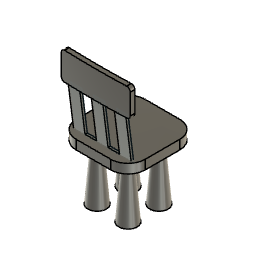
Chair (Autodesk Fusion 360 design; units mm, degrees)
Autodesk Fusion 360 part; units mm, degrees
note: some values were not read from the file. Chosen so that the rebuilt part matches the saved one: which face or edge a step refers to. Set by a fixed rule: which sketch regions a step uses.
sketch "Sketch1" plane through (0, 0, 0) normal (0, 0, 1) x (1, 0, 0)
  line L0 (0, 0) -> (20, 0)
  line L1 (0, 0) -> (0, 250)
  spline S0 degree 5 poles (0, 250) (1.763, 249.8564) (5.2208, 249.5461) (10.2027, 249.0117) (16.4289, 248.1586) (23.4627, 246.8396) (29.6575, 245.2376) (34.2312, 243.5585) (37.1499, 242.0595) (38.8803, 240.8979) (39.7703, 240.1911) (40, 240) knots 0 0 0 0 0 0 0.1 0.2 0.3 0.4 0.5 0.6 0.63638 0.63638 0.63638 0.63638 0.63638 0.63638
  line L2 (20, 0) -> (40, 240)
  dimension "d4" = 250
  dimension "d6" = 20
  constraint coincident L0.start L1.start
  constraint perpendicular L0 L1
  measures "d4" distance of L0.start L1.end
  measures "d6" distance of L0.start L0.end
revolve "Revolve1" add sketch "Sketch1" angle 360 about axis through (0, 0, 0) along (0, 1, 0) makes body 1
move_body "Move1" bodies 1 to x (1, 0, 0) y (0, 0, -1) z (0, 1, 0) at (0, 25, 250)
ref_plane "WorkPlane1" through (0, 120, 0) normal (0, 1, 0) x (0, 0, 1)
sketch "Sketch2" plane through (0, 120, 0) normal (0, 1, 0) x (1, 0, 0)
pattern_circular "C-Pattern1" count 4 over 360 about axis through (0, 120, 0) along (0, 0, 1) of bodies 1 makes body 2 at (78.3678, 154.5371, 30) makes body 3 at (-34.5371, 198.3678, 30) makes body 4 at (-68.9267, 91.8997, 30)
sketch "Sketch3" plane through (0, 0, 250) normal (0, 0, 1) x (-1, 0, 0)
  circle A0 centre (0, -215) radius 20
  line L0 (106.1582, -225.9737) -> (0.1845, -332.132)
  line L1 (106.1582, -225.9737) -> (212.132, -119.8155)
  line L2 (212.132, -119.8155) -> (-0.1845, 92.132)
  line L3 (-0.1845, 92.132) -> (-212.132, -120.1845)
  line L4 (-212.132, -120.1845) -> (0.1845, -332.132)
  constraint perpendicular L1 L2
  constraint perpendicular L2 L3
  constraint perpendicular L0 L4
extrude "Extrude1" add sketch "Sketch3" along normal blind 40 contours A0 | L0 L1 L2 L3 L4 bodies 1 2 3 4
fillet "Fillet1" radius 75 1 edges at (0.1845, -92.132, 270) on bodies 1
fillet "Fillet2" radius 75 1 edges at (212.132, 120.1845, 270) on bodies 1
fillet "Fillet3" radius 75 1 edges at (-0.1845, 332.132, 270) on bodies 1
fillet "Fillet4" radius 75 1 edges at (-212.132, 119.8155, 270) on bodies 1
ref_plane "WorkPlane2" through (88.4652, 31.6886, 270) normal (0.707722, -0.706491, 0) x (0.706491, 0.707722, 0)
sketch "Sketch4" plane through (28.4653, -28.4158, 0) normal (0.707722, -0.706491, 0) x (0.706491, 0.707722, 0)
  line L0 (-65, 275) -> (-25, 275)
  line L1 (-25, 275) -> (-15, 275)
  line L2 (-15, 275) -> (-25, 275)
  line L3 (-25, 275) -> (-50, 470)
  line L4 (-50, 470) -> (-40, 470)
  line L5 (-40, 470) -> (-15, 275)
  dimension "d25" = 40
  dimension "d26" = 10
  dimension "d27" = 10
  constraint horizontal L0
  constraint parallel L0 L1
  constraint horizontal L2
  constraint horizontal L4
  measures "d25" distance of L0.start L0.end
  measures "d26" distance of L0.end L1.end
  measures "d27" distance of L1.end L0.end
extrude "Extrude2" add sketch "Sketch4" against normal blind 250 separate body makes body 5
ref_plane "WorkPlane3" through (-79.4284, 40.4333, 372.5) normal (0.700756, 0.701976, 0.127164) x (0.08984, 0.089997, -0.991882)
sketch "Sketch5" plane through (14.0796, 14.1041, 2.555) normal (0.700756, 0.701976, 0.127164) x (0.08984, 0.089997, -0.991882)
ref_plane "WorkPlane4" through (0, 120, 290) normal (0, 0, 1) x (1, 0, 0)
sketch "Sketch6" plane through (0, 0, 290) normal (0, 0, 1) x (1, 0, 0)
move_body "Move2" bodies 5 1 to x (0.707107, 0.707107, 0) y (-0.707107, 0.707107, 0) z (0, 0, 1) at (84.8528, 35.1472, 0)
sketch "Sketch7" plane through (0, 0, 290) normal (0, 0, 1) x (-1, 0, 0)
  arc A0 (149.9347, -44.8695) -> (74.8695, 30.0652) centre (74.9347, -44.9348) ccw
  line L0 (74.8695, 30.0652) -> (-75.1305, 29.9347)
  arc A1 (-75.1305, 29.9347) -> (-150.0652, -45.1305) centre (-75.0652, -45.0653) ccw
  line L1 (-150.0652, -45.1305) -> (-149.9347, -195.1305)
  arc A2 (-149.9347, -195.1305) -> (-74.8695, -270.0652) centre (-74.9347, -195.0652) ccw
  line L2 (-74.8695, -270.0652) -> (75.1305, -269.9347)
  arc A3 (75.1305, -269.9347) -> (150.0652, -194.8695) centre (75.0652, -194.9347) ccw
  line L3 (150.0652, -194.8695) -> (149.9347, -44.8695)
  line L4 (-125, -50) -> (-75, -49.9565)
  line L5 (-75, -49.9565) -> (-25, -49.913)
  line L6 (-25, -49.913) -> (24.9999, -49.8695)
  line L7 (24.9999, -49.8695) -> (74.9999, -49.826)
  line L8 (74.9999, -49.826) -> (124.9999, -49.7825)
  line L9 (-75, -49.9565) -> (-25, -49.9565)
  line L10 (-25, -49.9565) -> (-25, 21.5768)
  line L11 (-25, 21.5768) -> (-75, 21.5768)
  line L12 (-75, 21.5768) -> (-75, -49.9565)
  line L13 (24.9999, -49.8695) -> (74.9999, -49.8695)
  line L14 (74.9999, -49.8695) -> (74.9999, 17.9113)
  line L15 (74.9999, 17.9113) -> (24.9999, 17.9113)
  line L16 (24.9999, 17.9113) -> (24.9999, -49.8695)
  dimension "d44" = 50
  dimension "d45" = 50
  dimension "d46" = 50
  dimension "d47" = 50
  dimension "d48" = 50
  dimension "d49" = 50
  dimension "d50" = 50
  constraint perpendicular L1 L4
  constraint parallel L4 L5
  constraint parallel L5 L6
  constraint parallel L5 L7
  constraint parallel L7 L8
  constraint horizontal L9
  constraint vertical L10
  constraint horizontal L11
  constraint vertical L12
  constraint horizontal L13
  constraint vertical L14
  constraint horizontal L15
  constraint vertical L16
  measures "d44" distance of L4.start L4.end
  measures "d45" distance of L4.end L5.end
  measures "d46" distance of L5.end L6.end
  measures "d47" distance of L6.end L7.end
  measures "d48" distance of L7.end L8.end
  measures "d49" distance of L4.end L9.end
  measures "d50" distance of L6.end L13.end
extrude "Extrude3" cut sketch "Sketch7" along normal blind 195 contours L5 L10 L11 L12 | L7 L14 L15 L16 bodies 5
sketch "Sketch8" plane through (-0.0474, 54.435, 6.9789) normal (-0.000863, 0.991881, 0.127164) x (-1, -0.00087, 0)
  line L0 (-24.9957, 466.8109) -> (-25.0158, 285.3376)
  line L1 (-25.0158, 285.3376) -> (-75.0158, 285.3376)
  line L2 (-75.0158, 285.3376) -> (-74.9958, 466.8109)
  line L3 (-74.9958, 466.8109) -> (-125.1044, 466.8109)
  line L4 (-125.1044, 466.8109) -> (-125.1044, 270.2148)
  line L5 (-125.1044, 270.2148) -> (124.8956, 270.2148)
  line L6 (124.8956, 270.2148) -> (124.8956, 466.8109)
  line L7 (124.8956, 466.8109) -> (75.0043, 466.8109)
  line L8 (75.0043, 466.8109) -> (74.9842, 285.3376)
  line L9 (74.9842, 285.3376) -> (24.9842, 285.3376)
  line L10 (24.9842, 285.3376) -> (25.0042, 466.8109)
  line L11 (25.0042, 466.8109) -> (-24.9957, 466.8109)
sketch "Sketch9" plane through (0, 0, 470) normal (0, 0, 1) x (-1, 0, 0)
  line L0 (-25, 14.9049) -> (-25, 4.9049)
  line L1 (-25, 4.9049) -> (24.9999, 4.9484)
  line L2 (24.9999, 4.9484) -> (24.9999, 14.9484)
  line L3 (24.9999, 14.9484) -> (-25, 14.9049)
  line L4 (-125, 15) -> (-125, 20)
  line L5 (-125, 20) -> (-125, 0)
  line L6 (125, 15) -> (125, 20)
  line L7 (125, 20) -> (125, 0)
  line L8 (-125, 0) -> (-150, 0)
  line L9 (-150, 0) -> (-150, 20)
  line L10 (125, 0) -> (150, 0)
  line L11 (150, 0) -> (150, 20)
  spline S0 degree 5 poles (-150, 0) (-144, 0.2252) (-132, 0.6558) (-114, 1.2428) (-90, 1.9056) (-60, 2.5206) (-30, 2.903) (0, 3.0339) (30, 2.903) (60, 2.5206) (90, 1.9056) (114, 1.2428) (132, 0.6558) (144, 0.2252) (150, 0) knots 0 0 0 0 0 0 0.1 0.2 0.3 0.4 0.5 0.6 0.7 0.8 0.9 1 1 1 1 1 1
  spline S1 degree 5 poles (-150, 20) (-144, 20.2252) (-132, 20.6558) (-114, 21.2428) (-90, 21.9056) (-60, 22.5206) (-30, 22.903) (0, 23.0339) (30, 22.903) (60, 22.5206) (90, 21.9056) (114, 21.2428) (132, 20.6558) (144, 20.2252) (150, 20) knots 0 0 0 0 0 0 0.1 0.2 0.3 0.4 0.5 0.6 0.7 0.8 0.9 1 1 1 1 1 1
  point P0 (0, 2.9687)
  point P1 (0, 22.9687)
  dimension "d57" = 5
  dimension "d58" = 20
  dimension "d59" = 5
  dimension "d60" = 20
  constraint parallel L4 L5
  constraint vertical L6
  constraint parallel L6 L7
  constraint perpendicular L5 L8
  constraint perpendicular L8 L9
  constraint perpendicular L7 L10
  constraint perpendicular L10 L11
  measures "d57" distance of L4.start L4.end
  measures "d58" distance of L4.end L5.end
  measures "d59" distance of L6.start L6.end
  measures "d60" distance of L6.end L7.end
extrude "Extrude4" add sketch "Sketch9" along normal blind 120 contours L0 L1 L2 L3 | L9 L11 S0 S1 bodies 5
fillet "Fillet5" radius 15 1 edges at (-150, -10, 470) on bodies 5
fillet "Fillet6" radius 15 1 edges at (-150, -10, 590) on bodies 5
fillet "Fillet7" radius 15 1 edges at (150, -10, 590) on bodies 5
fillet "Fillet8" radius 15 1 edges at (150, -10, 470) on bodies 5
